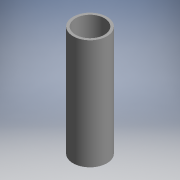
# Autodesk Inventor part: LZ80_Rohr_Schubstange90
Saved by Autodesk Inventor 2021 (Build 250183000, 183)
## iProperties
Part Number: LZ80_Rohr_Schubstange90
Material: Generic
Catalog Web Link: www.cadenas.de
Description: LZ80 Rohr Schubstange-Bauteil LZ80
Vendor: ROSEKRIEGER
Document SubType Name: Modeling
Designer: partserver
Manufacturer: ROSEKRIEGER
Mass: 45.3332 g
Surface Area: 309.196 cm^2
Volume: 45.3332 cm^3
Density: 1 g/cm^3
Appearance: PSOLRGB-192-192-192
Category: PARTsolutions
Company: ROSEKRIEGER
PSOL_IDENT_0: {$CADENAS_DATA\23d-libs\rose_krieger\linearkomponenten\pool_lineartechnik\_hubsaeule_zyliinder\elekt
PSOL_IDENT_1: rozylinder\elekzyl_lz80\lz80_rohr_schubstange.prj},207 {VTYP=3D},{NB=LZ80_Rohr_Schubstange90},{LINA=
PSOL_IDENT_2: LZ80_Rohr_Schubstange90},{NN=LZ80 Rohr Schubstange},{DATE=02.12.2020 11:16:41},{GEOMDATE=16.10.2013
PSOL_IDENT_3: 11:37:39},{VERSION=},{LINEID=10},{WBVAR=HUB},{WBNUMERIC=HUB}  {NB=LZ80_Rohr_Schubstange90},{LINA=LZ8
PSOL_IDENT_4: 0_Rohr_Schubstange90},{KT=DUMMY},{IDNR=},{ARTIKEL=LZ80_Rohr_Schubstange},{AUSDURCH=40.000},{INDURCH=
PSOL_IDENT_5: 34.000},{GRUNDLAE=311.000},{HUB=90},{YHUB=[7.5:202.5/7.5]},{RF=1.000}
NB: LZ80_Rohr_Schubstange90
NN: LZ80 Rohr Schubstange
NT: Bauteil LZ80
NBSYN: $ARTIKEL.$HUB.
LINA: LZ80_Rohr_Schubstange90
CATALOG: RK Rose+Krieger
ARTIKEL: LZ80_Rohr_Schubstange
AUSDURCH: 40
INDURCH: 34
GRUNDLAE: 311
HUB: 90
RF: 1
SUPPLIER: ROSEKRIEGER
ARTICLENO: LZ80_Rohr_Schubstange90
BOMINFO: LZ80_Rohr_Schubstange90
CREATOR: CADENAS GmbH
Title: LZ80_Rohr_Schubstange90
Author: Cadenas PARTsolutions
Comments: Bauteil LZ80
Autodesk Inventor part; units mm, degrees
sketch "Skizze_1" plane through (0, 0, 0) normal (0, 0, 1) x (1, 0, 0)
  circle A0 centre (0, 0) radius 20
  circle A1 centre (0, 0) radius 17
  constraints: 2 centre point
extrude "Extrusion1" add sketch "Skizze_1" along normal blind 130
ref_plane "EPROHR_XY" through (0, 0, 0) normal (0, 0, 1) x (1, 0, 0)
ref_plane "EPROHR_YZ" through (0, 0, 0) normal (1, 0, 0) x (0, 1, 0)
ref_plane "EPROHR_ZX" through (0, 0, 0) normal (0, 1, 0) x (0, 0, 1)
body "Solid1"
